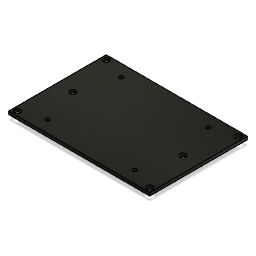
площадка rasberri v1 (Autodesk Fusion 360 design; units mm, degrees)
Autodesk Fusion 360 part; units mm, degrees
sketch "Sketch1" plane through (0, 0, 0) normal (0, 1, 0) x (1, 0, 0)
  line L0 (-70, -50) -> (-12, -50)
  line L1 (-12, -50) -> (-12, -1)
  line L2 (-12, -1) -> (-70, -1)
  line L3 (-70, -1) -> (-70, -50)
  circle A0 centre (-70, -50) radius 1.35
  circle A1 centre (-12, -50) radius 1.35
  circle A2 centre (-70, -1) radius 1.35
  circle A3 centre (-12, -1) radius 1.35
  line L4 (-41, -50) -> (-41, -25.5)
  line L5 (0, -53) -> (-82, -53)
  line L6 (-82, -53) -> (-82, 2)
  line L7 (-82, 2) -> (0, 2)
  line L8 (0, 2) -> (0, -53)
  line L9 (0, -53) -> (-82, 2) construction
  line L10 (-82, -53) -> (0, 2) construction
  circle A4 centre (-77.6409, -25.5) radius 2
  circle A5 centre (-4.3591, -25.5) radius 2
  point P0 (-41, -25.5)
  dimension "d1" = 58
  dimension "d2" = 49
  dimension "d3" = 2.7
  dimension "d4" = 2.7
  dimension "d5" = 2.7
  dimension "d6" = 2.7
  dimension "d7" = 4
  constraint horizontal L0
  constraint vertical L1
  constraint horizontal L2
  constraint vertical L3
  constraint coincident L0.start L3.end
  constraint coincident L0.end L1.start
  constraint coincident L2.end L3.start
  constraint coincident L1.end L2.start
  constraint midpoint L0 L4.start
  constraint perpendicular L0 L4
  constraint horizontal L5
  constraint perpendicular L5 L6
  constraint parallel L5 L7
  constraint parallel L6 L8
  constraint coincident L9 P0
  constraint coincident L10 P0
  constraint coincident P0 L4.end
  constraint symmetric L4 A4 A5
  measures "d1" distance of L0.start L0.end
  measures "d2" distance of L0.start L2.end
  measures "d3" diameter of A0
  measures "d4" diameter of A1
  measures "d5" diameter of A2
  measures "d6" diameter of A3
  measures "d7" diameter of A4
extrude "Extrude1" add sketch "Sketch1" along normal blind 2 contours L0 L1 L2 L3 A0 A1 A2 A3 | L5 L6 L7 L8
sketch "Sketch2" plane through (0, 0, 0) normal (0, -1, 0) x (1, 0, 0)
  circle A0 centre (-4.3591, 25.5) radius 2
  circle A1 centre (-70, 50) radius 1.35
  circle A2 centre (-77.6409, 25.5) radius 2
  circle A3 centre (-12, 50) radius 1.35
  circle A4 centre (-70, 1) radius 1.35
  circle A5 centre (-12, 1) radius 1.35
  line L0 (-82, -2) -> (0, -2)
  line L1 (0, -2) -> (0, 53)
  line L2 (0, 53) -> (-82, 53)
  line L3 (-82, 53) -> (-82, -2)
  circle A6 centre (-12, 50) radius 3
  circle A7 centre (-12, 50) radius 1.35
  circle A8 centre (-12, 1) radius 1.35
  circle A9 centre (-12, 1) radius 2
  circle A10 centre (-70, 1) radius 1.35
  circle A11 centre (-70, 1) radius 2
  circle A12 centre (-70, 50) radius 1.35
  circle A13 centre (-70, 50) radius 2
  circle A14 centre (-12, 50) radius 2
  dimension "d10" = 4
  dimension "d11" = 4
  dimension "d12" = 4
  constraint concentric A3 A6
  constraint tangent L2 A6
  constraint concentric A3 A7
  constraint concentric A5 A8
  constraint concentric A8 A9
  constraint concentric A4 A10
  constraint concentric A10 A11
  constraint concentric A1 A12
  constraint concentric A12 A13
  constraint concentric A6 A14
  measures "d10" diameter of A11
  measures "d11" diameter of A13
  measures "d12" diameter of A14
extrude "Extrude2" add sketch "Sketch2" along normal blind 3 contours A9 | A11 | A13 | A14
extrude "Extrude3" add 1 faces at (0, 0.6667, 16.3333) along direction (1, 0, 0) blind 6
extrude "Extrude4" add 1 faces at (-82, 0.6667, 34.6667) along direction (-1, 0, 0) blind 6
extrude "Extrude5" add 1 faces at (-25.3333, 0.6667, -2) along direction (0, 0, -1) blind 5
extrude "Extrude6" add 1 faces at (-25.3333, 0.6667, 53) along direction (0, 0, 1) blind 5
sketch "Sketch3" plane through (0, 0, 0) normal (0, -1, 0) x (1, 0, 0)
  circle A0 centre (-12, 1) radius 2
  circle A1 centre (-12, 50) radius 2
  circle A2 centre (-70, 1) radius 2
  circle A3 centre (-70, 50) radius 2
  circle A4 centre (-4.3591, 25.5) radius 2
  circle A5 centre (-77.6409, 25.5) radius 2
  line L0 (6, -7) -> (6, 58)
  line L1 (6, 58) -> (-88, 58)
  line L2 (-88, 58) -> (-88, -7)
  line L3 (-88, -7) -> (6, -7)
  circle A6 centre (-85, 55) radius 2
  line L4 (-41, 58) -> (-41, 35)
  line L5 (-88, 25.5) -> (-67.9088, 25.5)
  circle A7 centre (3, 55) radius 2
  circle A8 centre (-85, -4) radius 2
  circle A9 centre (3, -4) radius 2
  constraint midpoint L1 L4.start
  constraint perpendicular L1 L4
  constraint midpoint L2 L5.start
  constraint perpendicular L2 L5
  constraint symmetric A6 L4 A7
  constraint symmetric A6 L5 A8
  constraint symmetric L5 A7 A9
extrude "Extrude7" cut sketch "Sketch3" against normal blind 15 contours A6 | A7 | A8 | A9
